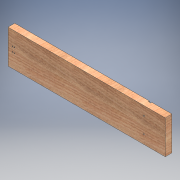
# Autodesk Inventor part: Base
Saved by Autodesk Inventor 2018 (Build 220112000, 112)
## iProperties
Created: 2019-05-10
Part Number: Base
Material: Generic
Document SubType Name: Modeling
Designer: aal_9
Density: 1 g/cm^3
Appearance: Default
Author: aal_9
Autodesk Inventor part; units mm, degrees
ref_plane "YZ Plane" through (0, 0, 0) normal (1, 0, 0) x (0, 1, 0)
ref_plane "XZ Plane" through (0, 0, 0) normal (0, 1, 0) x (-1, 0, 0)
ref_plane "XY Plane" through (0, 0, 0) normal (0, 0, 1) x (1, 0, 0)
sketch "Sketch1" plane through (0, 0, 0) normal (0, 1, 0) x (-1, 0, 0)
  line L0 (0, 0) -> (700, 0)
  line L1 (700, 0) -> (700, -150)
  line L2 (700, -150) -> (0, -150)
  line L3 (0, -150) -> (0, 0)
  dimension "d0" = 700
  dimension "d1" = 150
  constraints: 8 end point, 2 parallel, 1 horizontal, 1 perpendicular
  measures "d0" distance of L1.end L2.end
  measures "d1" distance of L0.end L1.end
extrude "Extrusion1" add sketch "Sketch1" along normal blind 30
sketch "Sketch2" plane through (0, 30, 0) normal (0, 1, 0) x (1, 0, 0)
  line L0 (-684, 59) -> (-668, 59)
  line L1 (-668, 59) -> (-668, 69)
  line L2 (-668, 69) -> (-684, 69)
  line L3 (-684, 69) -> (-684, 59)
  line L4 (-700, 150) -> (-700, 0) projected
  line L5 (-700, 75) -> (-334.1666, 75) construction
  line L6 (-684, 91) -> (-668, 91)
  line L7 (-668, 91) -> (-668, 81)
  line L8 (-668, 81) -> (-684, 81)
  line L9 (-684, 81) -> (-684, 91)
  point P0 (0, 0)
  dimension "d4" = 6
  dimension "d5" = 16
  dimension "d6" = 16
  dimension "d7" = 10
  constraints: 18 end point, 4 symmetric about line, 2 horizontal, 2 parallel, 1 midpoint, 1 perpendicular
  measures "d4" distance between parallel lines of L2 L5
  measures "d5" distance between parallel lines of L4 L3
  measures "d6" distance of L0.start L0.end
  measures "d7" distance of L0.end L1.end
extrude "Extrusion2" cut sketch "Sketch2" against normal blind 5
sketch "Sketch4" plane through (0, 30, 0) normal (0, 1, 0) x (1, 0, 0)
  line L0 (-100, 150) -> (-90, 150)
  line L1 (-90, 150) -> (-90, 0)
  line L2 (-90, 0) -> (-100, 0)
  line L3 (-100, 0) -> (-100, 150)
  line L4 (-700, 150) -> (-700, 0) projected
  line L5 (0, 150) -> (-700, 150) projected
  point P0 (0, 0)
  dimension "d10" = 600
  dimension "d11" = 10
  dimension "d14" = 0
  constraints: 8 end point, 2 parallel, 1 horizontal, 1 perpendicular
  measures "d10" distance between parallel lines of L4 L3
  measures "d11" distance of L1.end L2.end
  measures "d14" distance between parallel lines of L5 L0
extrude "Extrusion3" cut sketch "Sketch4" against normal blind 5
sketch "Sketch5" plane through (0, 0, 0) normal (0, -1, 0) x (1, 0, 0)
  line L0 (-90, -150) -> (-90, 0) projected
  line L1 (-700, -150) -> (0, -150) projected
  line L2 (0, 0) -> (-700, 0) projected
  point P0 (-95, -40)
  point P1 (-95, -110)
  dimension "d15" = 5
  dimension "d16" = 5
  dimension "d17" = 40
  dimension "d18" = 40
  measures "d15" distance from line of L0 point (-95, -40)
  measures "d16" distance from line of L0 point (-95, -110)
  measures "d17" distance from line of L1 point (-95, -110)
  measures "d18" distance from line of L2 point (-95, -40)
hole "Hole1" at (-95, 0, -40) at (-95, 0, -110) direction (0, 1, 0) diameter 3 end through all counterbore diameter 5 counterbore depth 3
sketch "Sketch6" plane through (0, 0, 0) normal (0, -1, 0) x (1, 0, 0)
  line L0 (-668, -59) -> (-684, -59) projected
  line L1 (-684, -69) -> (-668, -69) projected
  line L2 (-668, -81) -> (-684, -81) projected
  line L3 (-684, -91) -> (-668, -91) projected
  line L4 (-684, -81) -> (-684, -91) projected
  line L5 (-668, -91) -> (-668, -81) projected
  line L6 (-684, -59) -> (-684, -69) projected
  line L7 (-668, -69) -> (-668, -59) projected
  point P0 (0, 0)
  point P1 (-680, -86)
  point P2 (-672, -86)
  point P3 (-672, -64)
  point P4 (-680, -64)
  dimension "d26" = 5
  dimension "d27" = 5
  dimension "d28" = 5
  dimension "d29" = 5
  dimension "d30" = 4
  dimension "d31" = 4
  dimension "d32" = 4
  dimension "d33" = 4
  measures "d26" distance from line of L0 point (-680, -64)
  measures "d27" distance from line of L1 point (-672, -64)
  measures "d28" distance from line of L2 point (-680, -86)
  measures "d29" distance from line of L3 point (-672, -86)
  measures "d30" distance from line of L4 point (-680, -86)
  measures "d31" distance from line of L5 point (-672, -86)
  measures "d32" distance from line of L6 point (-680, -64)
  measures "d33" distance from line of L7 point (-672, -64)
hole "Hole2" at (-680, 0, -86) at (-672, 0, -86) at (-672, 0, -64) at (-680, 0, -64) direction (0, 1, 0) diameter 3 end through all counterbore diameter 4 counterbore depth 2
body "Solid1"
